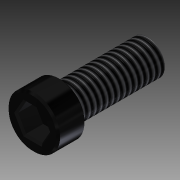
# Autodesk Inventor part: Gearbox Hex Machine Screw 4
Saved by Autodesk Inventor 2013 (Build 170138000, 138)
## iProperties
Created: 2012-03-30
Part Number: Gearbox Hex Machine Screw 4
Material: Steel
Document SubType Name: Modeling
Designer: Moses
Mass: 5.54917 g
Surface Area: 6.91401 cm^2
Volume: 0.7069 cm^3
Density: 7.85 g/cm^3
Author: Moses
Autodesk Inventor part; units mm, degrees
ref_plane "YZ Plane" through (0, 0, 0) normal (1, 0, 0) x (0, 1, 0)
ref_plane "XZ Plane" through (0, 0, 0) normal (0, 1, 0) x (-1, 0, 0)
ref_plane "XY Plane" through (0, 0, 0) normal (0, 0, 1) x (1, 0, 0)
sketch "Sketch1" plane through (0, 0, 0) normal (0, 0, 1) x (1, 0, 0)
  circle A0 centre (0, 0) radius 3.4925
  circle A1 centre (0, 0) radius 2.3495
  line L0 (2.1997, 0) -> (1.0999, -1.905)
  line L1 (1.0999, -1.905) -> (-1.0999, -1.905)
  line L2 (-1.0999, -1.905) -> (-2.1997, 0)
  line L3 (-2.1997, 0) -> (-1.0999, 1.905)
  line L4 (-1.0999, 1.905) -> (1.0999, 1.905)
  line L5 (1.0999, 1.905) -> (2.1997, 0)
  dimension "d0" = 6.985
  dimension "d1" = 4.699
  dimension "d2" = 3.81
  constraints: 12 end point, 3 coincident, 2 centre point, 1 horizontal, 13 other
  measures "d0" diameter of A0
  measures "d1" diameter of A1
  measures "d2" distance between parallel lines of L1 L4
extrude "Extrusion1" add sketch "Sketch1" along normal blind 3.81 contours A0 | A1
extrude "Extrusion2" add sketch "Sketch1" against normal blind 11.811 contours A1 | L0 L1 L2 L3 L4 L5
extrude "Extrusion3" add sketch "Sketch1" along normal blind 1.27 contours L0 L1 L2 L3 L4 L5
thread "Thread1" size "10-32 UNF" class "2A" standard "ANSI Unified Screw Threads" full length
chamfer "Chamfer1" distance 0.254 angle 45 8 edges at (-3.4925, 0, 3.81) (-3.4925, 0, 0) (-1.6498, 0.9525, 3.81) (-1.6498, -0.9525, 3.81) (0, -1.905, 3.81) (1.6498, -0.9525, 3.81) (1.6498, 0.9525, 3.81) (0, 1.905, 3.81)
body "Solid1"
